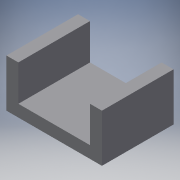
# Autodesk Inventor part: To Next Termination
Saved by Autodesk Inventor 2016 (Build 200138000, 138)
## iProperties
Created: 2013-12-03
Part Number: To Next Termination
Material: Generic
Document SubType Name: Modeling
Designer: John
Density: 1 g/cm^3
Appearance: Default
Author: John
Autodesk Inventor part; units mm, degrees
ref_plane "YZ Plane" through (0, 0, 0) normal (1, 0, 0) x (0, 1, 0)
ref_plane "XZ Plane" through (0, 0, 0) normal (0, 1, 0) x (-1, 0, 0)
ref_plane "XY Plane" through (0, 0, 0) normal (0, 0, 1) x (1, 0, 0)
sketch "Sketch1" plane through (0, 0, 0) normal (0, 0, 1) x (1, 0, 0)
  line L0 (0, 0) -> (50.8, 0)
  line L1 (50.8, 0) -> (50.8, 25.4)
  line L2 (50.8, 25.4) -> (0, 25.4)
  line L3 (0, 25.4) -> (0, 0)
  dimension "d0" = 50.8
  dimension "d1" = 25.4
  constraints: 8 end point, 2 parallel, 1 horizontal, 1 perpendicular
  measures "d0" distance of L2.end L1.end
  measures "d1" distance of L1.end L0.end
extrude "Extrusion1" add sketch "Sketch1" along normal blind 38.1
sketch "Sketch2" plane through (0, 0, 38.1) normal (0, 0, 1) x (1, 0, 0)
  line L0 (0, 0) -> (50.8, 0) projected
  line L1 (50.8, 0) -> (50.8, 25.4) projected
  line L2 (50.8, 25.4) -> (0, 25.4) projected
  line L3 (0, 25.4) -> (0, 0) projected
  line L4 (6.35, 25.4) -> (44.45, 25.4)
  line L5 (44.45, 25.4) -> (44.45, 6.35)
  line L6 (44.45, 6.35) -> (6.35, 6.35)
  line L7 (6.35, 6.35) -> (6.35, 25.4)
  dimension "d4" = 6.35
  dimension "d5" = 6.35
  dimension "d6" = 6.35
  constraints: 8 end point, 2 parallel, 1 horizontal, 1 perpendicular, 1 point on line
  measures "d4" distance between parallel lines of L1 L5
  measures "d5" distance between parallel lines of L0 L6
  measures "d6" distance between parallel lines of L3 L7
extrude "Extrusion2" cut sketch "Sketch2" against normal through all contours L2 L5 L6 L7
equation "\"d5\" = d4"
equation "\"d6\" = d4"
body "Solid1"
